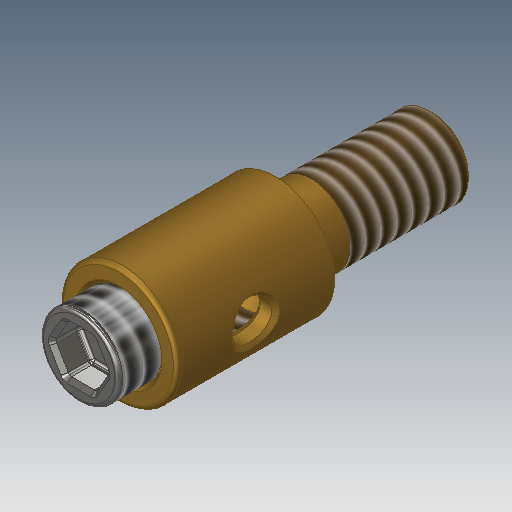
# Autodesk Inventor part: C-04-0
Saved by Autodesk Inventor 2019 (Build 230136000, 136)
## iProperties
Created: 2022-04-09
Part Number: C-04-0
Material: Brass, Soft Yellow
Document SubType Name: Modeling
Designer: solyo
Density: 8.47 g/cm^3
Appearance: Brass - Satin
Mass: 0.319251 g
Surface Area: 1.23187 cm^2
Volume: 0.037692 cm^3
Author: solyo
Autodesk Inventor part; units mm, degrees
ref_plane "YZ Plane" through (0, 0, 0) normal (1, 0, 0) x (0, 1, 0)
ref_plane "XZ Plane" through (0, 0, 0) normal (0, 1, 0) x (-1, 0, 0)
ref_plane "XY Plane" through (0, 0, 0) normal (0, 0, 1) x (1, 0, 0)
sketch "Sketch1" plane through (0, 0, 0) normal (0, 0, 1) x (1, 0, 0)
  circle A0 centre (0, 0) radius 1
  dimension "d0" = 2
  constraints: 1 centre point, 1 coincident
  measures "d0" diameter of A0
extrude "Extrusion1" add sketch "Sketch1" along normal blind 4
sketch "Sketch2" plane through (0, 0, 4) normal (0, 0, 1) x (1, 0, 0)
  circle A0 centre (0, 0) radius 1.5
  dimension "d3" = 3
  constraints: 1 centre point, 1 coincident
  measures "d3" diameter of A0
extrude "Extrusion2" add sketch "Sketch2" along normal blind 4
fillet "Fillet1" radius 0.1 1 edges at (-1.5, 0, 8)
sketch "Sketch3" plane through (0, 0, 0) normal (1, 0, 0) x (0, 1, 0)
  circle A0 centre (0, 6) radius 0.5
  line L0 (1.5, 7.9) -> (-1.5, 7.9) projected
  point P0 (0, 0)
  point P1 (-1.5, 4.1)
  point P2 (1.5, 4.1)
  dimension "d12" = 1.9
  dimension "d14" = 1
  constraints: 1 centre point, 1 vertical alignment
  measures "d12" distance from line of L0 A0.centre
  measures "d14" diameter of A0
extrude "Extrusion3" cut sketch "Sketch3" along normal through all both and the other way through all
sketch "Sketch4" plane through (0, 0, 8) normal (0, 0, 1) x (1, 0, 0)
  point P0 (0, 0)
  point P1 (0, 0)
  constraints: 1 coincident
hole "Hole1" at (0, 0, 8) direction (0, 0, -1) diameter 2.013 depth 3.2 tip angle 118 thread size "M2.5x0.45" class "6H" standard "ISO Metric profile"
chamfer "Chamfer2" distance 0.1 angle 45 8 edges at (-1, 0, 0) (1.4142, -0.5, 6) (1.4567, 0.3579, 6.3491) (1.4567, 0.3579, 5.6509) (-1.4142, -0.5, 6) (0.8735, -0.5, 6) (-0.8735, -0.5, 6) (0, 1.0065, 8)
sketch "Sketch5" plane through (0, 0, 8) normal (0, 0, 1) x (1, 0, 0)
  circle A0 centre (0, 0) radius 1.0065 projected
extrude "Extrusion4" add sketch "Sketch5" along normal blind 1 and the other way blind 2 separate body
thread "Thread3" size "M2.2x0.45" class "6g" standard "ANSI Metric M Profile" full length
sketch "Sketch6" plane through (0, 0, 9) normal (0, 0, 1) x (1, 0, 0)
  line L0 (-0.35, 0.6062) -> (0.35, 0.6062)
  line L1 (0.35, 0.6062) -> (0.7, 0)
  line L2 (0.7, 0) -> (0.35, -0.6062)
  line L3 (0.35, -0.6062) -> (-0.35, -0.6062)
  line L4 (-0.35, -0.6062) -> (-0.7, 0)
  line L5 (-0.7, 0) -> (-0.35, 0.6062)
  circle A0 centre (0, 0) radius 1.0065 projected
  point P0 (0, 0.6062)
  dimension "d36" = 120
  dimension "d37" = 120
  dimension "d38" = 0.7
  constraints: 12 end point, 4 equal length, 2 parallel, 1 horizontal, 1 horizontal alignment, 1 midpoint, 1 vertical alignment
  measures "d36" angle of L0 L5
  measures "d37" angle of L4 L5
  measures "d38" distance of L0.start L0.end
extrude "Extrusion5" cut sketch "Sketch6" against normal blind 0.7 contours L0 L1 L2 L3 L4 L5 bodies 2
fillet "Fillet3" radius 0.1 14 edges at (0.35, 0.6062, 8.65) (-0.35, 0.6062, 8.65) (-0.7, 0, 8.65) (-0.35, -0.6062, 8.65) (0.35, -0.6062, 8.65) (0.7, 0, 8.65) (-1.0065, 0, 9) (-1.0065, 0, 6) (-0.525, -0.3031, 8.3) (-0.525, 0.3031, 8.3) (0, 0.6062, 8.3) (0.525, 0.3031, 8.3) (0.525, -0.3031, 8.3) (0, -0.6062, 8.3)
chamfer "Chamfer3" distance 0.1 angle 45 12 edges at (0, 0.6062, 9) (0.3423, 0.5928, 9) (0.525, 0.3031, 9) (0.6845, 0, 9) (0.525, -0.3031, 9) (0.3423, -0.5928, 9) (0, -0.6062, 9) (-0.3423, -0.5928, 9) (-0.525, -0.3031, 9) (-0.6845, 0, 9) (-0.525, 0.3031, 9) (-0.3423, 0.5928, 9)
thread "Thread4" size "M2x0.4" class "6g" standard "ANSI Metric M Profile" length 3
equation "\"d12\" = d13"
equation "\"d37\" = d36"
equation "\"d13\" = 1.9"
body "Solid1"
body "Solid2"
